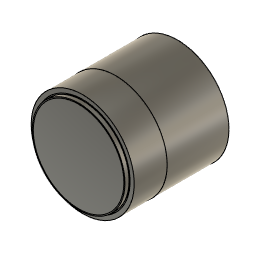
beamdump (Autodesk Fusion 360 design; units mm, degrees)
Autodesk Fusion 360 part; units mm, degrees
sketch "Sketch1" plane through (0, 0, 0) normal (0, 0, 1) x (1, 0, 0) in component "lejek"
  line L0 (0, 0) -> (25, 0)
  line L1 (25, 0) -> (25, 30)
  line L2 (25, 30) -> (0, 0)
  line L3 (0, 80) -> (0, -63.8211) construction
  dimension "d1" = 25
  dimension "d2" = 30
  constraint coincident L0.start L2.end
  constraint horizontal L0
  constraint perpendicular L0 L1
  constraint perpendicular L0 L3
  measures "d1" distance of L0.start L0.end
  measures "d2" distance of L0.end L1.end
revolve "Revolve1" add sketch "Sketch1" angle 360 about axis through (0, 80, 0) along (0, -1, 0) makes body 1 in component "lejek"
sketch "Sketch2" plane through (0, 0, 0) normal (0, -1, 0) x (1, 0, 0) in component "lejek"
  circle A0 centre (0, 0) radius 25
  circle A1 centre (0, 0) radius 2.5
  dimension "d4" = 5
  constraint concentric A0 A1
  measures "d4" diameter of A1
extrude "Extrude1" cut sketch "Sketch2" against normal blind 10 contours A1 bodies 1 in component "lejek"
sketch "Sketch1 (2)" plane through (0, 0, 0) normal (0, 1, 0) x (1, 0, 0) in component "koncowka"
  circle A0 centre (0, 0) radius 25
  constraint coincident A0.centre origin
extrude "Extrude1'" add sketch "Sketch1 (2)" along normal blind 16 separate body makes body 2 in component "koncowka"
sketch "Sketch2 (2)" plane through (0, 0, 0) normal (0, 1, 0) x (1, 0, 0) in component "koncowka"
  circle A0 centre (0, 0) radius 2.5
  dimension "d9" = 5
  constraint coincident A0.centre origin
  measures "d9" diameter of A0
extrude "Extrude3" cut sketch "Sketch2 (2)" along normal up to surface (16 mm away) bodies 2 in component "koncowka"
sketch "Sketch3" plane through (0, 0, 0) normal (0, -1, 0) x (1, 0, 0) in component "koncowka"
  circle A0 centre (0, 0) radius 2.5
  circle A1 centre (0, 0) radius 25
  circle A2 centre (0, 0) radius 22
  dimension "d15" = -3
extrude "Extrude4" cut sketch "Sketch3" against normal blind 13 contours A2 bodies 2 in component "koncowka"
sketch "Sketch4" plane through (0, 0, 0) normal (0, -1, 0) x (1, 0, 0) in component "koncowka"
  circle A0 centre (0, 0) radius 22
  circle A1 centre (0, 0) radius 25
  circle A2 centre (0, 0) radius 23
  dimension "d18" = 1
extrude "Extrude5" cut sketch "Sketch4" against normal blind 1 contours A2 bodies 2 in component "koncowka"
sketch "Sketch5" plane through (0, 16, 0) normal (0, 1, 0) x (-1, 0, 0) in component "koncowka"
  circle A0 centre (0, 0) radius 2.5
  circle A1 centre (0, 0) radius 25
  circle A2 centre (15, 0) radius 1.5
  dimension "d22" = 3
  measures "d22" diameter of A2
extrude "Extrude6" add sketch "Sketch5" along normal blind 3 contours A2 bodies 2 in component "koncowka"
sketch "Sketch6" plane through (0, 16, 0) normal (0, 1, 0) x (-1, 0, 0) in component "koncowka"
  circle A0 centre (15, 0) radius 1.5
  circle A1 centre (0, 0) radius 2.5
  circle A2 centre (0, 0) radius 25
  circle A3 centre (0, 15) radius 1.5
  circle A4 centre (-15, 0) radius 1.5
  circle A5 centre (0, -15) radius 1.5
  dimension "d26" = 360
extrude "Extrude8" add sketch "Sketch6" along normal blind 3 contours A4 bodies 2 in component "koncowka"
extrude "Extrude7" add sketch "Sketch6" along normal blind 3 contours A3 bodies 2 in component "koncowka"
sketch "Sketch7" plane through (0, 16, 0) normal (0, 1, 0) x (-1, 0, 0) in component "koncowka"
  circle A0 centre (0, 15) radius 1.5
  circle A1 centre (15, 0) radius 1.5
  circle A2 centre (0, 0) radius 2.5
  circle A3 centre (0, 0) radius 25
  circle A4 centre (-15, 0) radius 1.5
extrude "Extrude9" add sketch "Sketch6" along normal blind 3 contours A5 bodies 2 in component "koncowka"
sketch "Sketch8" plane through (0, 0, 0) normal (0, -1, 0) x (1, 0, 0) in component "koncowka"
  circle A0 centre (0, 0) radius 2.5
  circle A1 centre (0, 0) radius 25
  circle A2 centre (0, 0) radius 22.9534
  constraint concentric A0 A2
sketch "Sketch3 (2)" plane through (0, 0, 0) normal (0, -1, 0) x (1, 0, 0) in component "lejek"
  circle A0 centre (0, 0) radius 2.5
  circle A1 centre (0, 0) radius 25
  circle A2 centre (15, -0.1245) radius 1.5
  circle A3 centre (0.1245, 15) radius 1.5
  circle A4 centre (-15, 0.1245) radius 1.5
  circle A5 centre (-0.1245, -15) radius 1.5
  dimension "d33" = 3
  dimension "d34" = 15
  dimension "d36" = 360
  measures "d33" diameter of A2
  measures "d34" horizontal distance of A0.centre A2.centre
extrude "Extrude2" cut sketch "Sketch3 (2)" against normal blind 3 contours A2 | A3 | A4 | A5 bodies 1 in component "lejek"
sketch "Sketch1 (3)" plane through (0, 0, 0) normal (0, 1, 0) x (1, 0, 0) in component "pokrywka"
  circle A0 centre (0, 0) radius 22
  circle A1 centre (0, 0) radius 22.5
  dimension "d39" = 44
  dimension "d40" = 45
  constraint coincident A0.centre A1.centre
  measures "d39" diameter of A0
  measures "d40" diameter of A1
extrude "Extrude2'" add sketch "Sketch1 (3)" along normal blind 4 separate body contours A0 makes body 3 in component "pokrywka"
extrude "Extrude1''" add sketch "Sketch1 (3)" along normal blind 2 separate body makes body 4 in component "pokrywka"
component "lejek" placed x (1, 0, 0) y (0, 1, 0) z (0, 0, 1) at (0, 0, 0)
component "koncowka" placed x (1, 0, 0) y (0, 1, 0) z (0, 0, 1) at (0, 0, 0)
component "pokrywka" placed x (1, 0, 0) y (0, 1, 0) z (0, 0, 1) at (0, 0, 0)
